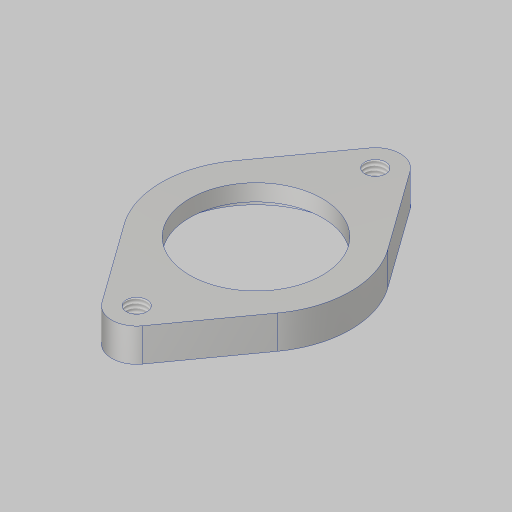
# Autodesk Inventor part: Retainer
Saved by Autodesk Inventor 2023.5 (Build 275446000, 446)
## iProperties
Created: 2025-01-25
Part Number: Retainer
Material: Aluminum 6061
Document SubType Name: Modeling
Designer: slick
Density: 2.7 g/cm^3
Appearance: Aluminum - Flat
Author: slick
Autodesk Inventor part; units mm, degrees
ref_plane "YZ Plane" through (0, 0, 0) normal (1, 0, 0) x (0, 1, 0)
ref_plane "XZ Plane" through (0, 0, 0) normal (0, 1, 0) x (-1, 0, 0)
ref_plane "XY Plane" through (0, 0, 0) normal (0, 0, 1) x (1, 0, 0)
sketch "Sketch1" plane through (0, 0, 0) normal (0, 1, 0) x (-1, 0, 0)
  circle A0 centre (0, 0) radius 12.7
  circle A1 centre (0, 0) radius 18.0975
  circle A2 centre (0, 22.86) radius 4.7625 construction
  circle A3 centre (0, -22.86) radius 4.7625 construction
  line L0 (3.8683, 25.6381) -> (14.6994, 10.5569)
  line L1 (-3.8683, 25.6381) -> (-14.6994, 10.5569)
  line L2 (-14.6994, -10.5569) -> (-3.8683, -25.6381)
  line L3 (3.8683, -25.6381) -> (14.6994, -10.5569)
  arc A4 (14.6994, -10.5569) -> (14.6994, 10.5569) centre (0, 0) ccw
  arc A5 (-3.8683, -25.6381) -> (3.8683, -25.6381) centre (0, -22.86) ccw
  arc A6 (-14.6994, 10.5569) -> (-14.6994, -10.5569) centre (0, 0) ccw
  arc A7 (3.8683, 25.6381) -> (-3.8683, 25.6381) centre (0, 22.86) ccw
  circle A8 centre (0, 0) radius 16.51
  dimension "d0" = 25.4
  dimension "d1" = 36.195
  dimension "d2" = 9.525
  dimension "d7" = 33.02
  constraints: 16 point on circle, 10 tangent, 9 centre point, 9 coincident, 8 end point, 3 equal radius, 2 vertical alignment
  measures "d0" diameter of A0
  measures "d1" diameter of A1
  measures "d2" diameter of A2
  measures "d7" diameter of A8
extrude "Extrusion1" add sketch "Sketch1" along normal blind 6.35 contours A1 | A1 L1 A7 L0 | L3 A5 L2 A1 | A8
extrude "Extrusion2" cut sketch "Sketch1" along normal blind 3.175 contours A8
hole "Hole1" at (0, 0, 22.86) at (0, 0, -22.86) direction (0, 1, 0) diameter 3.9624 end through all thread size "10-32 UNF" class "2B" standard "ANSI Unified Screw Threads"
body "Solid1"
